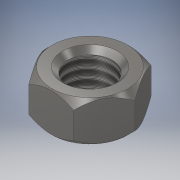
# Autodesk Inventor part: Porca sextavada 1 quarto
Saved by Autodesk Inventor 2019.4 (Build 234330000, 330)
## iProperties
Created: 2021-04-26
Part Number: Porca sextavada 1 quarto
Material: Aço, carbono
Document SubType Name: Modeling
Designer: Lattes
Density: 7.85 g/cm^3
Appearance: Semipolido
Author: Lattes
Autodesk Inventor part; units mm, degrees
ref_plane "YZ Plane" through (0, 0, 0) normal (1, 0, 0) x (0, 1, 0)
ref_plane "XZ Plane" through (0, 0, 0) normal (0, 1, 0) x (-1, 0, 0)
ref_plane "XY Plane" through (0, 0, 0) normal (0, 0, 1) x (1, 0, 0)
sketch "Esboço1" plane through (0, 0, 0) normal (0, 1, 0) x (-1, 0, 0)
  circle A0 centre (0, 0) radius 3.175
  line L0 (-3.2072, -5.555) -> (-6.4144, 0)
  line L1 (-6.4144, 0) -> (-3.2072, 5.555)
  line L2 (-3.2072, 5.555) -> (3.2072, 5.555)
  line L3 (3.2072, 5.555) -> (6.4144, 0)
  line L4 (6.4144, 0) -> (3.2072, -5.555)
  line L5 (3.2072, -5.555) -> (-3.2072, -5.555)
  dimension "d0" = 6.35
  constraints: 12 end point, 2 coincident, 1 centre point, 13 other
  measures "d0" diameter of A0
extrude "Extrusão1" add sketch "Esboço1" along normal blind 5.74
thread "Rosca1" size "1/4-20 UNC" class "2B" standard "ANSI Unified Screw Threads" full length
sketch "Esboço2" plane through (0, 0, 0) normal (0, 0, 1) x (1, 0, 0)
  line L0 (0, 0) -> (-3.175, 0)
  line L1 (3.2072, 5.74) -> (-3.2072, 5.74) projected
  line L2 (-3.2072, 5.74) -> (-6.4144, 5.74) projected
  line L3 (0, 0) -> (0, 10.6611)
  line L4 (-6.4144, 4.74) -> (-5.4144, 5.74)
  line L5 (-3.175, 4.99) -> (-3.925, 5.74)
  line L6 (-3.2072, 2.87) -> (-11.6119, 2.87)
  line L7 (-6.4144, 4.74) -> (-6.4144, 5.74)
  line L8 (-6.4144, 5.74) -> (-5.4144, 5.74)
  line L9 (-3.925, 5.74) -> (-3.175, 5.74)
  line L10 (-3.175, 4.99) -> (-3.175, 5.74)
  line L11 (-3.2072, 0) -> (-6.4144, 0)
  line L12 (-6.4144, 1) -> (-5.4144, 0)
  line L13 (-3.175, 0.75) -> (-3.925, 0)
  line L14 (-6.4144, 1) -> (-6.4144, 0)
  line L15 (-6.4144, 0) -> (-5.4144, 0)
  line L16 (-3.925, 0) -> (-3.175, 0)
  line L17 (-3.175, 0.75) -> (-3.175, 0)
  line L18 (-6.4144, 0) -> (-3.2072, 0) projected
  line L19 (-6.4144, 0) -> (-5.4144, 0)
  point P0 (-3.175, 5.74)
  dimension "d6" = 1
  dimension "d7" = 1
  dimension "d8" = 0.75
  dimension "d9" = 0.75
  constraints: 34 end point, 6 symmetric about line, 2 collinear, 2 vertical, 1 horizontal, 1 perpendicular, 1 point on line
  measures "d6" distance of L4.start L2.end
  measures "d7" distance of L4.end L2.end
  measures "d8" distance of L5.start L9.end
  measures "d9" distance of L5.end L9.end
revolve "Revolução1" cut sketch "Esboço2" angle 360 about axis through (0, 0, 0) along (0, 1, 0)
equation "\"d7\" = d6"
equation "\"d9\" = d8"
